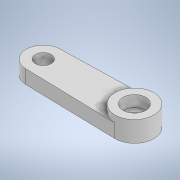
# Autodesk Inventor part: eje de servo 1
Saved by Autodesk Inventor 2021 (Build 250183000, 183)
## iProperties
Created: 2021-03-31
Part Number: eje de servo 1
Material: Generic
Document SubType Name: Modeling
Designer: trejo
Density: 1 g/cm^3
Appearance: Default
Author: trejo
Autodesk Inventor part; units mm, degrees
ref_plane "YZ Plane" through (0, 0, 0) normal (1, 0, 0) x (0, 1, 0)
ref_plane "XZ Plane" through (0, 0, 0) normal (0, 1, 0) x (-1, 0, 0)
ref_plane "XY Plane" through (0, 0, 0) normal (0, 0, 1) x (1, 0, 0)
sketch "Sketch1" plane through (0, 0, 0) normal (0, 1, 0) x (-1, 0, 0)
  line L0 (0, 0) -> (10, 0) construction
  circle A0 centre (10, 0) radius 3.75
  circle A1 centre (10, 0) radius 1.75
  line L1 (0, 0) -> (-10, 0) construction
  circle A2 centre (-10, 0) radius 4.25
  line L2 (10.0938, 3.7488) -> (-9.8938, 4.2487)
  line L3 (10.0938, -3.7488) -> (-9.8938, -4.2487)
  dimension "d1" = 7.5
  dimension "d0" = 10
  dimension "d2" = 3.5
  dimension "d3" = 10
  constraints: 8 end point, 2 coincident, 2 horizontal, 2 symmetric about line, 1 centre point, 8 other
  measures "d0" distance of L0.start L0.end
  measures "d2" diameter of A1
  measures "d3" distance of L0.start L1.end
extrude "Extrusion1" add sketch "Sketch1" along normal mid plane 3
sketch "Sketch2" plane through (0, 1.5, 0) normal (0, 1, 0) x (1, 0, 0)
  arc A0 (9.8938, -4.2487) -> (9.8938, 4.2487) centre (10, 0) ccw projected
  circle A1 centre (10, 0) radius 2.5
  circle A2 centre (10, 0) radius 4.25
  point P0 (0, 0)
  point P1 (9.8937, 4.2487)
  point P2 (9.8938, -4.2487)
  dimension "d9" = 5
  constraints: 2 centre point, 2 coincident, 1 concentric
  measures "d9" diameter of A1
extrude "Extrusion2" add sketch "Sketch2" along normal blind 1.5
sketch "Sketch4" plane through (10, 1.5, 0) normal (0, 1, 0) x (1, 0, 0)
  circle A0 centre (0, 0) radius 2.5 projected
  circle A1 centre (0, 0) radius 2.5
  point P0 (-10, 0)
  dimension "d13" = 5
  constraints: 1 centre point, 1 coincident
  measures "d13" diameter of A1
extrude "Extrusion3" cut sketch "Sketch4" against normal blind 1
sketch "Sketch5" plane through (10, 0.5, 0) normal (0, 1, 0) x (1, 0, 0)
  circle A0 centre (0, 0) radius 2.5 projected
  circle A1 centre (0, 0) radius 1.25
  point P0 (-10, 0)
  dimension "d16" = 2.5
  constraints: 1 centre point, 1 coincident
  measures "d16" diameter of A1
extrude "Extrusion4" cut sketch "Sketch5" against normal blind 0.8 contours A1
sketch "Sketch6" plane through (0, -1.5, 0) normal (0, -1, 0) x (1, 0, 0)
  arc A0 (9.8938, -4.2487) -> (9.8938, 4.2487) centre (10, 0) ccw projected
  circle A1 centre (10, 0) radius 2.5
  point P0 (0, 0)
  dimension "d19" = 5
  constraints: 1 centre point, 1 coincident
  measures "d19" diameter of A1
extrude "Extrusion5" cut sketch "Sketch6" against normal blind 1.2
body "Solid1"
